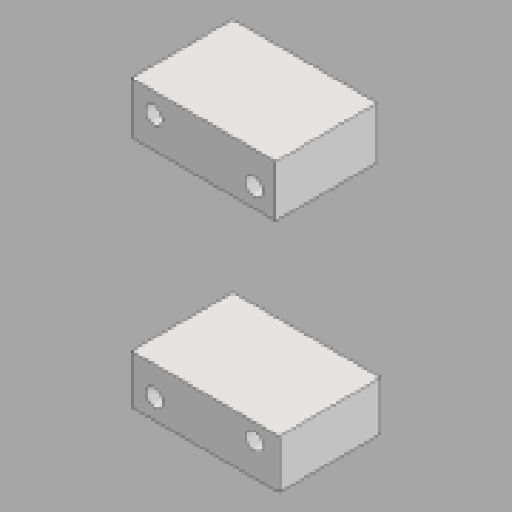
# Autodesk Inventor part: Подставка
Saved by Autodesk Inventor 2025 (Build 290162000, 162)
## iProperties
Created: 2025-04-10
Part Number: Подставка
Material: Типовые
Document SubType Name: Modeling
Designer: Artem Sannikov
Density: 1 g/cm^3
Appearance: По умолчанию
Author: Artem Sannikov
Autodesk Inventor part; units mm, degrees
ref_plane "YZ Plane" through (0, 0, 0) normal (1, 0, 0) x (0, 1, 0)
ref_plane "XZ Plane" through (0, 0, 0) normal (0, 1, 0) x (-1, 0, 0)
ref_plane "XY Plane" through (0, 0, 0) normal (0, 0, 1) x (1, 0, 0)
sketch "Эскиз1" plane through (0, 0, 0) normal (0, 0, 1) x (1, 0, 0)
  line L0 (15.5244, 128.0541) -> (-30.4166, 128.0541)
  line L1 (-30.4166, 128.0541) -> (-30.4166, 111.7143)
  line L2 (-30.4166, 111.7143) -> (15.5244, 111.7143)
  line L3 (15.5244, 111.7143) -> (15.5244, 128.0541)
  line L4 (16.5668, 52.9885) -> (-30.3753, 52.9885)
  line L5 (-30.3753, 52.9885) -> (-30.3753, 37.5067)
  line L6 (-30.3753, 37.5067) -> (16.5668, 37.5067)
  line L7 (16.5668, 37.5067) -> (16.5668, 52.9885)
  point P0 (0, 0)
  constraints: 16 end point, 4 parallel, 2 horizontal, 2 perpendicular
extrude "Выдавливание1" add sketch "Эскиз1" along normal blind 32.25
sketch "Эскиз2" plane through (0, 0, 32.25) normal (0, 0, 1) x (1, 0, 0)
  circle A0 centre (8.5875, 117.7715) radius 2.75 projected
  circle A1 centre (-23.2502, 121.4735) radius 2.75 projected
  circle A2 centre (-23.0424, 43.8992) radius 2.75 projected
  circle A3 centre (8.775, 47.7717) radius 2.75 projected
  point P0 (0, 0)
extrude "Выдавливание2" cut sketch "Эскиз2" against normal blind 32.25
